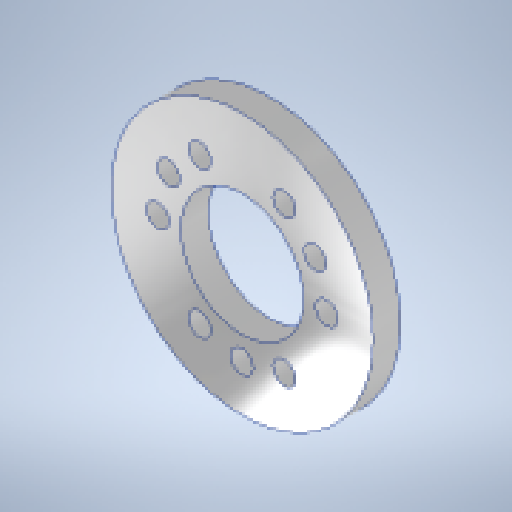
# Autodesk Inventor part: base_plate2
Saved by Autodesk Inventor 2024 (Build 280153000, 153)
## iProperties
Created: 2025-02-13
Part Number: base_plate2
Material: アルミニウム 6061
Document SubType Name: Modeling
Designer: tanoue_kota
Density: 2.7 g/cm^3
Appearance: アルミニウム - フラット
Author: tanoue_kota
Autodesk Inventor part; units mm, degrees
ref_plane "YZ Plane" through (0, 0, 0) normal (1, 0, 0) x (0, 1, 0)
ref_plane "XZ Plane" through (0, 0, 0) normal (0, 1, 0) x (-1, 0, 0)
ref_plane "XY Plane" through (0, 0, 0) normal (0, 0, 1) x (1, 0, 0)
sketch "スケッチ1" plane through (0, 0, 0) normal (0, 0, 1) x (1, 0, 0)
  circle A0 centre (0, 0) radius 23.5
  dimension "d0" = 47
  constraints: 1 centre point, 1 coincident
  measures "d0" diameter of A0
extrude "押し出し1" add sketch "スケッチ1" along normal blind 5
sketch "スケッチ2" plane through (0, 0, 5) normal (0, 0, 1) x (1, 0, 0)
  line L0 (0, 0) -> (0, -15.18)
  circle A0 centre (0, 0) radius 15.18
  line L1 (0, 0) -> (7.59, -13.1463)
  point P0 (13.1463, 7.59)
  point P1 (-13.1463, 7.59)
  point P2 (15.18, 0)
  point P3 (7.59, 13.1463)
  point P4 (-7.59, 13.1463)
  point P5 (-15.18, 0)
  point P6 (-7.59, -13.1463)
  dimension "d3" = 30.36
  dimension "d6" = 360
  dimension "d8" = 30
  dimension "d11" = 360
  constraints: 4 end point, 3 coincident, 2 point on circle, 1 centre point, 1 vertical, 11 other
  measures "d3" diameter of A0
  measures "d8" angle of L0 L1
hole "穴1" at (0, -15.18, 5) at (13.1463, 7.59, 5) at (-13.1463, 7.59, 5) at (7.59, -13.1463, 5) at (15.18, 0, 5) at (7.59, 13.1463, 5) at (-7.59, 13.1463, 5) at (-15.18, 0, 5) at (-7.59, -13.1463, 5) direction (0, 0, -1) diameter 4.1 end through all
sketch "スケッチ3" plane through (0, 0, 5) normal (0, 0, 1) x (1, 0, 0)
  circle A0 centre (0, 0) radius 11
  dimension "d20" = 22
  constraints: 1 centre point, 1 coincident
  measures "d20" diameter of A0
extrude "押し出し2" cut sketch "スケッチ3" against normal blind 5
